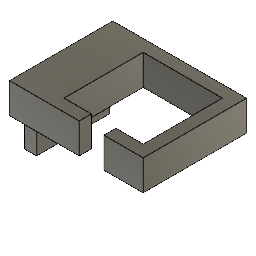
assembly v3 (Autodesk Fusion 360 archive; units mm, degrees)
design "holder_L"
Autodesk Fusion 360 part; units mm, degrees
sketch "Sketch1" plane through (0, 0, 0) normal (0, 0, 1) x (1, 0, 0)
  line L0 (0, 0) -> (13, 0)
  line L1 (13, 0) -> (13, 13)
  line L2 (13, 13) -> (0, 13)
  line L3 (0, 13) -> (0, 0)
  line L4 (-2, -2) -> (15, -2)
  line L5 (15, -2) -> (15, 15)
  line L6 (15, 15) -> (-2, 15)
  line L7 (-2, 15) -> (-2, -2)
  dimension "d1" = 13
  dimension "d2" = 13
  dimension "d3" = 2
  constraint horizontal L0
  constraint vertical L1
  constraint horizontal L2
  constraint vertical L3
  constraint coincident L0.start L3.end
  measures "d1" distance of L1.end L2.end
  measures "d2" distance of L0.end L1.end
extrude "Extrude1" add sketch "Sketch1" along normal blind 5
sketch "Sketch2" plane through (0, 0, 0) normal (0, 1, 0) x (-1, 0, 0)
  line L0 (-13, 0) -> (0, 0)
  line L1 (0, 0) -> (0, 5)
  line L2 (0, 5) -> (-13, 5)
  line L3 (-13, 5) -> (-13, 0)
  line L4 (-8.5, 5) -> (-4.5, 5)
  line L5 (-4.5, 5) -> (-4.5, 0)
  line L6 (-4.5, 0) -> (-8.5, 0)
  line L7 (-8.5, 0) -> (-8.5, 5)
  line L8 (-6.5, 0) -> (-6.5, 5)
  dimension "d6" = 4
  dimension "d7" = 90
  constraint horizontal L4
  constraint vertical L5
  constraint horizontal L6
  constraint vertical L7
  constraint coincident L0 L5.end
  constraint coincident L2 L4.start
  constraint midpoint L6 L8.start
  constraint midpoint L2 L8.end
  measures "d6" distance of L4.start L4.end
  measures "d7" angle of L4 L8
extrude "Extrude2" cut sketch "Sketch2" against normal blind 10 contours L0 L2 L4 L6 L7 L8 | L0 L2 L4 L5 L6 L8
extrude "Extrude3" add 1 faces at (-2, 9.3333, 1.6667) along direction (-1, 0, 0) blind 5
sketch "Sketch3" plane through (0, 0, 0) normal (0, 0, -1) x (1, 0, 0)
  line L0 (8.5, 2) -> (8.5, 0)
  line L1 (8.5, 0) -> (13, 0)
  line L2 (13, 0) -> (13, -13)
  line L3 (13, -13) -> (0, -13)
  line L4 (0, -13) -> (0, 0)
  line L5 (0, 0) -> (4.5, 0)
  line L6 (4.5, 0) -> (4.5, 2)
  line L7 (4.5, 2) -> (-7, 2)
  line L8 (-7, 2) -> (-7, -15)
  line L9 (-7, -15) -> (15, -15)
  line L10 (15, -15) -> (15, 2)
  line L11 (15, 2) -> (8.5, 2)
  line L12 (-7, 2) -> (-5, 2)
  line L13 (-5, 2) -> (-5, -15)
  line L14 (-5, -15) -> (-7, -15)
  line L15 (-7, -15) -> (-7, 2)
  dimension "d12" = 2
  constraint horizontal L12
  constraint vertical L13
  constraint horizontal L14
  constraint vertical L15
  constraint coincident L9 L13.end
  constraint coincident L7.end L8.start
  measures "d12" distance of L7.end L12.end
extrude "Extrude4" add sketch "Sketch3" along normal blind 6 contours L7 L8 L9 L12 L13 L14 L15
sketch "Sketch4" plane through (-5, 0, 0) normal (1, 0, 0) x (0, 1, 0)
  line L0 (15, 0) -> (-2, 0)
  line L1 (-2, 0) -> (-2, -6)
  line L2 (-2, -6) -> (15, -6)
  line L3 (15, -6) -> (15, 0)
  line L4 (-2, -2) -> (15, -2)
  circle A0 centre (3.5, -2) radius 1.5
  circle A1 centre (9.5, -2) radius 1.5
  line L5 (3.5, -2) -> (9.5, -2)
  line L6 (6.5, -2) -> (6.5, 0)
  dimension "d15" = 2
  dimension "d16" = 3
  dimension "d17" = 3
  dimension "d18" = 6
  dimension "d19" = 90
  constraint coincident L1 L4.start
  constraint coincident L3 L4.end
  constraint perpendicular L3 L4
  constraint coincident L4 A0.centre
  constraint coincident L4 A1.centre
  constraint coincident A0.centre L5.start
  constraint coincident A1.centre L5.end
  constraint midpoint L5 L6.start
  constraint midpoint L0 L6.end
  measures "d15" distance of L0 L4
  measures "d16" diameter of A0
  measures "d17" diameter of A1
  measures "d18" distance of A0.centre A1.centre
  measures "d19" angle of L0 L6
extrude "Extrude5" cut sketch "Sketch4" against normal blind 5 contours L4 A1 L5 | L4 A1 L5 | L4 A0 L5 | L4 A0 L5
sketch "Sketch5" plane through (-5, 0, 0) normal (1, 0, 0) x (0, 1, 0)
  circle A0 centre (3.5, -2) radius 1.5
  circle A1 centre (9.5, -2) radius 1.5
  line L0 (15, 0) -> (-2, 0)
  line L1 (-2, 0) -> (-2, -6)
  line L2 (-2, -6) -> (15, -6)
  line L3 (15, -6) -> (15, 0)
  line L4 (0.5, 0) -> (12.5, 0)
  line L5 (12.5, 0) -> (12.5, -6)
  line L6 (12.5, -6) -> (0.5, -6)
  line L7 (0.5, -6) -> (0.5, 0)
  line L8 (-2, -6) -> (15, -6)
  line L9 (15, -6) -> (15, 0)
  line L10 (15, 0) -> (-2, 0)
  line L11 (-2, 0) -> (-2, -6)
  dimension "d22" = 3
  dimension "d23" = 3
  constraint horizontal L4
  constraint vertical L5
  constraint horizontal L6
  constraint vertical L7
  constraint coincident L2 L5.end
  constraint coincident L0 L4.start
  constraint horizontal L8
  constraint vertical L9
  constraint horizontal L10
  constraint vertical L11
  constraint coincident L0.start L3.end
  constraint coincident L1.end L2.start
  measures "d22" distance of A0.centre L7
  measures "d23" distance of A1.centre L5
extrude "Extrude6" cut sketch "Sketch5" against normal blind 5 contours L0 L2 L3 L5 L8 L9 L10 | L0 L1 L2 L7 L8 L10 L11

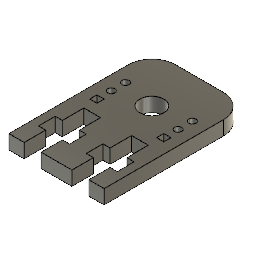
design "stand_L"
Autodesk Fusion 360 part; units mm, degrees
sketch "Sketch1" plane through (0, 0, 0) normal (0, 0, 1) x (1, 0, 0)
  line L0 (0, 0) -> (40, 0)
  line L1 (40, 0) -> (40, 60)
  line L2 (40, 60) -> (0, 60)
  line L3 (0, 60) -> (0, 0)
  line L4 (20, 60) -> (20, 27.089)
  circle A0 centre (20, 40) radius 5
  line L5 (6.5, 0) -> (13.5, 0)
  line L6 (13.5, 0) -> (13.5, 25)
  line L7 (13.5, 25) -> (6.5, 25)
  line L8 (6.5, 25) -> (6.5, 0)
  line L9 (26.5, 0) -> (33.5, 0)
  line L10 (33.5, 0) -> (33.5, 25)
  line L11 (33.5, 25) -> (26.5, 25)
  line L12 (26.5, 25) -> (26.5, 0)
  line L13 (10, 25) -> (30, 25)
  line L14 (20, 25) -> (20, 0)
  line L15 (0, 16) -> (40, 16)
  line L16 (3.5, 16) -> (16.5, 16)
  line L17 (16.5, 16) -> (16.5, 9)
  line L18 (16.5, 9) -> (3.5, 9)
  line L19 (3.5, 9) -> (3.5, 16)
  line L20 (3.5, 12.5) -> (6.5, 12.5)
  line L21 (10, 9) -> (10, 0)
  line L22 (23.5, 16) -> (23.5, 9)
  line L23 (23.5, 9) -> (36.5, 9)
  line L24 (36.5, 9) -> (36.5, 16)
  dimension "d1" = 40
  dimension "d2" = 60
  dimension "d3" = 10
  dimension "d4" = 40
  dimension "d5" = 7
  dimension "d6" = 7
  dimension "d7" = 25
  dimension "d8" = 25
  dimension "d9" = 20
  dimension "d10" = 90
  dimension "d11" = 90
  dimension "d12" = 13
  dimension "d13" = 90
  dimension "d14" = 7
  constraint horizontal L0
  constraint vertical L1
  constraint horizontal L2
  constraint vertical L3
  constraint coincident L0.start L3.end
  constraint midpoint L2 L4.start
  constraint perpendicular L2 L4
  constraint coincident L4 A0.centre
  constraint horizontal L5
  constraint vertical L6
  constraint horizontal L7
  constraint vertical L8
  constraint coincident L0 L5.start
  constraint horizontal L9
  constraint vertical L10
  constraint horizontal L11
  constraint vertical L12
  constraint coincident L0 L9.start
  constraint midpoint L7 L13.start
  constraint midpoint L11 L13.end
  constraint midpoint L13 L14.start
  constraint midpoint L0 L14.end
  constraint coincident L3 L15.start
  constraint coincident L1 L15.end
  constraint perpendicular L1 L15
  constraint horizontal L16
  constraint vertical L17
  constraint horizontal L18
  constraint vertical L19
  constraint coincident L15 L16.start
  constraint midpoint L19 L20.start
  constraint midpoint L8 L20.end
  constraint midpoint L18 L21.start
  constraint midpoint L5 L21.end
  constraint symmetric L14 L16.start L24.end
  constraint symmetric L14 L16.end L22.start
  constraint symmetric L14 L17.end L22.end
  constraint symmetric L14 L18.end L23.end
  measures "d1" distance of L0.start L0.end
  measures "d2" distance of L0.end L1.end
  measures "d3" diameter of A0
  measures "d4" distance of L0 A0.centre
  measures "d5" distance of L6.end L7.end
  measures "d6" distance of L10.end L11.end
  measures "d7" distance of L5.start L7.end
  measures "d8" distance of L9.end L10.end
  measures "d9" distance of L13.start L13.end
  measures "d10" angle of L0 L14
  measures "d11" angle of L8 L20
  measures "d12" distance of L17.end L18.end
  measures "d13" angle of L18 L21 L9.start
  measures "d14" distance of L16.end L17.end
extrude "Extrude1" add sketch "Sketch1" along normal blind 6 contours L0 L3 L8 L15 L18 L19 | L1 L2 L3 L7 L8 L10 L11 L13 L15 L16 | L0 L6 L14 L15 L17 L18 | L0 L12 L14 L15 L22 L23 | L6 L13 L14 L15 L16 | L12 L13 L14 L15 | L0 L1 L10 L15 L23 L24
sketch "Sketch2" plane through (0, 0, 6) normal (0, 0, 1) x (-1, 0, 0)
  circle A0 centre (-20, -40) radius 5
  line L0 (-33.5, 0) -> (-40, 0)
  line L1 (-40, 0) -> (-40, -60)
  line L2 (-40, -60) -> (0, -60)
  line L3 (0, -60) -> (0, 0)
  line L4 (0, 0) -> (-6.5, 0)
  line L5 (-6.5, 0) -> (-6.5, -9)
  line L6 (-6.5, -9) -> (-3.5, -9)
  line L7 (-3.5, -9) -> (-3.5, -16)
  line L8 (-3.5, -16) -> (-6.5, -16)
  line L9 (-6.5, -16) -> (-6.5, -25)
  line L10 (-6.5, -25) -> (-13.5, -25)
  line L11 (-13.5, -25) -> (-13.5, -16)
  line L12 (-13.5, -16) -> (-16.5, -16)
  line L13 (-16.5, -16) -> (-16.5, -9)
  line L14 (-16.5, -9) -> (-13.5, -9)
  line L15 (-13.5, -9) -> (-13.5, 0)
  line L16 (-13.5, 0) -> (-26.5, 0)
  line L17 (-26.5, 0) -> (-26.5, -9)
  line L18 (-26.5, -9) -> (-23.5, -9)
  line L19 (-23.5, -9) -> (-23.5, -16)
  line L20 (-23.5, -16) -> (-26.5, -16)
  line L21 (-26.5, -16) -> (-26.5, -25)
  line L22 (-26.5, -25) -> (-33.5, -25)
  line L23 (-33.5, -25) -> (-33.5, -16)
  line L24 (-33.5, -16) -> (-36.5, -16)
  line L25 (-36.5, -16) -> (-36.5, -9)
  line L26 (-36.5, -9) -> (-33.5, -9)
  line L27 (-33.5, -9) -> (-33.5, 0)
  line L28 (0, -40) -> (-40, -40)
  line L29 (-6, -45) -> (-6, -35)
  circle A1 centre (-6, -43) radius 1.5
  circle A2 centre (-6, -37) radius 1.5
  line L30 (-6, -43) -> (-6, -37)
  line L31 (-6, -40) -> (0, -40)
  line L32 (-20, -40) -> (-20, -45)
  circle A3 centre (-34, -43) radius 1.5
  circle A4 centre (-34, -37) radius 1.5
  dimension "d17" = 6
  dimension "d18" = 3
  dimension "d19" = 3
  dimension "d20" = 6
  dimension "d21" = 90
  constraint coincident L3 L28.start
  constraint coincident L1 L28.end
  constraint perpendicular L1 L28
  constraint perpendicular L28 L29
  constraint coincident L29 A1.centre
  constraint coincident L29 A2.centre
  constraint coincident A1.centre L30.start
  constraint coincident A2.centre L30.end
  constraint midpoint L30 L31.start
  constraint coincident A0.centre L32.start
  constraint coincident A0 L32.end
  constraint vertical L32
  constraint coincident L28 A0.centre
  constraint symmetric A1 L32 A3
  constraint symmetric A2 L32 A4
  measures "d17" distance of L3 L29
  measures "d18" diameter of A1
  measures "d19" diameter of A2
  measures "d20" distance of A1.centre A2.centre
  measures "d21" angle of L3 L31
extrude "Extrude2" cut sketch "Sketch2" against normal blind 5 contours L29 A1 L30 | L29 A1 L30 | L29 A2 L30 | L29 A2 L30 | A3 | A4
sketch "Sketch3" plane through (0, 0, 6) normal (0, 0, 1) x (-1, 0, 0)
  circle A0 centre (-6, -37) radius 1.5
  circle A1 centre (-34, -43) radius 1.5
  circle A2 centre (-6, -43) radius 1.5
  circle A3 centre (-34, -37) radius 1.5
  circle A4 centre (-20, -40) radius 5
  line L0 (-33.5, 0) -> (-40, 0)
  line L1 (-40, 0) -> (-40, -60)
  line L2 (-40, -60) -> (0, -60)
  line L3 (0, -60) -> (0, 0)
  line L4 (0, 0) -> (-6.5, 0)
  line L5 (-6.5, 0) -> (-6.5, -9)
  line L6 (-6.5, -9) -> (-3.5, -9)
  line L7 (-3.5, -9) -> (-3.5, -16)
  line L8 (-3.5, -16) -> (-6.5, -16)
  line L9 (-6.5, -16) -> (-6.5, -25)
  line L10 (-6.5, -25) -> (-13.5, -25)
  line L11 (-13.5, -25) -> (-13.5, -16)
  line L12 (-13.5, -16) -> (-16.5, -16)
  line L13 (-16.5, -16) -> (-16.5, -9)
  line L14 (-16.5, -9) -> (-13.5, -9)
  line L15 (-13.5, -9) -> (-13.5, 0)
  line L16 (-13.5, 0) -> (-26.5, 0)
  line L17 (-26.5, 0) -> (-26.5, -9)
  line L18 (-26.5, -9) -> (-23.5, -9)
  line L19 (-23.5, -9) -> (-23.5, -16)
  line L20 (-23.5, -16) -> (-26.5, -16)
  line L21 (-26.5, -16) -> (-26.5, -25)
  line L22 (-26.5, -25) -> (-33.5, -25)
  line L23 (-33.5, -25) -> (-33.5, -16)
  line L24 (-33.5, -16) -> (-36.5, -16)
  line L25 (-36.5, -16) -> (-36.5, -9)
  line L26 (-36.5, -9) -> (-33.5, -9)
  line L27 (-33.5, -9) -> (-33.5, 0)
  line L28 (0, -31) -> (-40, -31)
  line L29 (-4.5, -32.5) -> (-7.5, -32.5)
  line L30 (-7.5, -32.5) -> (-7.5, -29.5)
  line L31 (-7.5, -29.5) -> (-4.5, -29.5)
  line L32 (-4.5, -29.5) -> (-4.5, -32.5)
  line L33 (-6, -37) -> (0, -37)
  line L34 (-6, -37) -> (-6, -32.5)
  line L35 (-4.5, -31) -> (0, -31)
  line L36 (-20, -40) -> (-20, -43)
  line L37 (-35.5, -32.5) -> (-32.5, -32.5)
  line L38 (-32.5, -32.5) -> (-32.5, -29.5)
  line L39 (-35.5, -29.5) -> (-35.5, -32.5)
  line L40 (-32.5, -29.5) -> (-35.5, -29.5)
  dimension "d24" = 3
  dimension "d25" = 3
  dimension "d26" = 90
  dimension "d27" = 6
  dimension "d28" = 90
  constraint coincident L3 L28.start
  constraint coincident L1 L28.end
  constraint perpendicular L1 L28
  constraint horizontal L29
  constraint vertical L30
  constraint horizontal L31
  constraint vertical L32
  constraint coincident A0.centre L33.start
  constraint coincident L3 L33.end
  constraint perpendicular L3 L33
  constraint midpoint L29 L34.end
  constraint midpoint L32 L35.start
  constraint coincident A4.centre L36.start
  constraint vertical L36
  constraint symmetric L29.start L36 L37.start
  constraint symmetric L29.end L36 L37.end
  constraint symmetric L30.end L36 L38.end
  constraint symmetric L31.end L36 L39.start
  measures "d24" distance of L29.end L30.end
  measures "d25" distance of L30.end L31.end
  measures "d26" angle of L29 L34
  measures "d27" distance of L28 L33
  measures "d28" angle of L32 L35
extrude "Extrude3" cut sketch "Sketch3" against normal blind 5 contours L28 L29 L30 L32 | L28 L30 L31 L32 | L28 L37 L38 L39 | L28 L38 L39 L40
fillet "Fillet1" radius 10 1 edges at (0, 60, 3)
fillet "Fillet2" radius 10 1 edges at (40, 60, 3)
extrude "Extrude4" cut 6 faces at (6.8158, 43.2169, 1) (6.1827, 37.4654, 1) (5.5, 31.5, 1) (33.5, 30.5, 1) (33.9601, 37.4654, 1) (33.2997, 43.1474, 1) along direction (0, 0, -1) blind 5

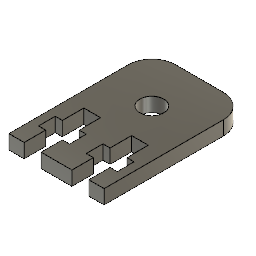
design "stand_R"
Autodesk Fusion 360 part; units mm, degrees
sketch "Sketch1" plane through (0, 0, 0) normal (0, 0, 1) x (1, 0, 0)
  line L0 (0, 0) -> (40, 0)
  line L1 (40, 0) -> (40, 60)
  line L2 (40, 60) -> (0, 60)
  line L3 (0, 60) -> (0, 0)
  line L4 (20, 60) -> (20, 27.089)
  circle A0 centre (20, 40) radius 5
  line L5 (6.5, 0) -> (13.5, 0)
  line L6 (13.5, 0) -> (13.5, 25)
  line L7 (13.5, 25) -> (6.5, 25)
  line L8 (6.5, 25) -> (6.5, 0)
  line L9 (26.5, 0) -> (33.5, 0)
  line L10 (33.5, 0) -> (33.5, 25)
  line L11 (33.5, 25) -> (26.5, 25)
  line L12 (26.5, 25) -> (26.5, 0)
  line L13 (10, 25) -> (30, 25)
  line L14 (20, 25) -> (20, 0)
  line L15 (0, 16) -> (40, 16)
  line L16 (3.5, 16) -> (16.5, 16)
  line L17 (16.5, 16) -> (16.5, 9)
  line L18 (16.5, 9) -> (3.5, 9)
  line L19 (3.5, 9) -> (3.5, 16)
  line L20 (3.5, 12.5) -> (6.5, 12.5)
  line L21 (10, 9) -> (10, 0)
  line L22 (23.5, 16) -> (23.5, 9)
  line L23 (23.5, 9) -> (36.5, 9)
  line L24 (36.5, 9) -> (36.5, 16)
  dimension "d1" = 40
  dimension "d2" = 60
  dimension "d3" = 10
  dimension "d4" = 40
  dimension "d5" = 7
  dimension "d6" = 7
  dimension "d7" = 25
  dimension "d8" = 25
  dimension "d9" = 20
  dimension "d10" = 90
  dimension "d11" = 90
  dimension "d12" = 13
  dimension "d13" = 90
  dimension "d14" = 7
  constraint horizontal L0
  constraint vertical L1
  constraint horizontal L2
  constraint vertical L3
  constraint coincident L0.start L3.end
  constraint midpoint L2 L4.start
  constraint perpendicular L2 L4
  constraint coincident L4 A0.centre
  constraint horizontal L5
  constraint vertical L6
  constraint horizontal L7
  constraint vertical L8
  constraint coincident L0 L5.start
  constraint horizontal L9
  constraint vertical L10
  constraint horizontal L11
  constraint vertical L12
  constraint coincident L0 L9.start
  constraint midpoint L7 L13.start
  constraint midpoint L11 L13.end
  constraint midpoint L13 L14.start
  constraint midpoint L0 L14.end
  constraint coincident L3 L15.start
  constraint coincident L1 L15.end
  constraint perpendicular L1 L15
  constraint horizontal L16
  constraint vertical L17
  constraint horizontal L18
  constraint vertical L19
  constraint coincident L15 L16.start
  constraint midpoint L19 L20.start
  constraint midpoint L8 L20.end
  constraint midpoint L18 L21.start
  constraint midpoint L5 L21.end
  constraint symmetric L14 L16.start L24.end
  constraint symmetric L14 L16.end L22.start
  constraint symmetric L14 L17.end L22.end
  constraint symmetric L14 L18.end L23.end
  measures "d1" distance of L0.start L0.end
  measures "d2" distance of L0.end L1.end
  measures "d3" diameter of A0
  measures "d4" distance of L0 A0.centre
  measures "d5" distance of L6.end L7.end
  measures "d6" distance of L10.end L11.end
  measures "d7" distance of L5.start L7.end
  measures "d8" distance of L9.end L10.end
  measures "d9" distance of L13.start L13.end
  measures "d10" angle of L0 L14
  measures "d11" angle of L8 L20
  measures "d12" distance of L17.end L18.end
  measures "d13" angle of L18 L21 L9.start
  measures "d14" distance of L16.end L17.end
extrude "Extrude1" add sketch "Sketch1" along normal blind 6 contours L0 L3 L8 L15 L18 L19 | L1 L2 L3 L7 L8 L10 L11 L13 L15 L16 | L0 L6 L14 L15 L17 L18 | L0 L12 L14 L15 L22 L23 | L6 L13 L14 L15 L16 | L12 L13 L14 L15 | L0 L1 L10 L15 L23 L24
fillet "Fillet1" radius 10 1 edges at (0, 60, 3)
fillet "Fillet2" radius 10 1 edges at (40, 60, 3)

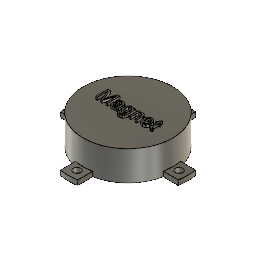
design "cap"
Autodesk Fusion 360 part; units mm, degrees
sketch "Sketch1" plane through (0, 0, 0) normal (0, 0, 1) x (1, 0, 0)
  circle A0 centre (0, 0) radius 16
  circle A1 centre (0, 0) radius 18
  dimension "d1" = 32
  dimension "d2" = 2
  constraint coincident A0.centre A1.centre
  constraint concentric A0 A1
  measures "d1" diameter of A0
  measures "d2" distance of A0 A1
extrude "Extrude1" add sketch "Sketch1" along normal blind 10
sketch "Sketch2" plane through (0, 0, 10) normal (0, 0, 1) x (-1, 0, 0)
  circle A0 centre (0, 0) radius 16
  circle A1 centre (0, 0) radius 18
  circle A2 centre (0, 0) radius 18
  constraint coincident A0.centre A1.centre
  constraint tangent A1 A2
extrude "Extrude2" add sketch "Sketch2" along normal blind 2 contours A0 | A1 A2
sketch "Sketch3" plane through (0, 0, 0) normal (0, 0, -1) x (1, 0, 0)
  circle A0 centre (0, 0) radius 16
  circle A1 centre (0, 0) radius 18
  line L0 (-3.5, 24) -> (3.5, 24)
  line L1 (3.5, 24) -> (3.5, -27)
  line L2 (3.5, -27) -> (-3.5, -27)
  line L3 (-3.5, -27) -> (-3.5, 24)
  line L4 (0, 0) -> (0, 18)
  line L5 (0, 18) -> (0, 24)
  circle A2 centre (0, 20.5) radius 1.5
  line L6 (0, 19) -> (0.9, 19)
  circle A3 centre (0, 0) radius 24
  line L7 (27, -3.5) -> (-24, -3.5)
  line L8 (-24, 3.5) -> (27, 3.5)
  circle A4 centre (-20.5, 0) radius 1.5
  line L9 (3.5, 27) -> (3.5, -24)
  line L10 (-3.5, -24) -> (-3.5, 27)
  circle A5 centre (0, -20.5) radius 1.5
  line L11 (-27, 3.5) -> (24, 3.5)
  line L12 (24, -3.5) -> (-27, -3.5)
  circle A6 centre (20.5, 0) radius 1.5
  dimension "d7" = 7
  dimension "d8" = 90
  dimension "d9" = 3
  dimension "d10" = 1
  dimension "d11" = 3.5
  dimension "d13" = 360
  constraint horizontal L0
  constraint vertical L1
  constraint horizontal L2
  constraint vertical L3
  constraint coincident A0.centre A1.centre
  constraint coincident A1 L4.end
  constraint parallel L1 L4
  constraint midpoint L0 L5.end
  constraint coincident L5 A2.centre
  constraint coincident A2 L6.start
  constraint coincident L5 L6.start
  constraint tangent A2 L6
  constraint coincident L5.end A3
  measures "d7" distance of L0.start L0.end
  measures "d8" angle of L0 L5
  measures "d9" diameter of A2
  measures "d10" distance of L4.end L6.start
  measures "d11" distance of L0 A2.centre
extrude "Extrude3" add sketch "Sketch3" against normal blind 3 contours A1 A3 L7 L8 L11 L12 | A1 L1 L5 A2 A3 L9 | A1 L1 L3 A3 L9 L10 | A1 L3 L5 A2 A3 L10 | A1 A3 L7 L8 L11 L12
extrude "Extrude4" cut 4 faces at (2.8333, -20.6333, 3) (-20.6707, 2.8319, 3) (20.6707, -2.8319, 3) (-2.8333, 20.6333, 3) along direction (0, 0, -1) blind 1
sketch "Sketch4" plane through (0, 0, 12) normal (0, 0, 1) x (-1, 0, 0)
  circle A0 centre (0, 0) radius 18
  line L0 (11, 2) -> (-11, 2) construction
  line L1 (-11, 2) -> (-11, -3) construction
  line L2 (-11, -3) -> (11, -3) construction
  line L3 (11, -3) -> (11, 2) construction
  dimension "d18" = 5
  text T0 "Magnet" font "Arial" height 5 align left top in box 22 x 5 at (11, 2) x (-1, 0) y (0, -1) spacing 1 kerned
extrude "Extrude5" add sketch "Sketch4" along normal blind 1 text T0

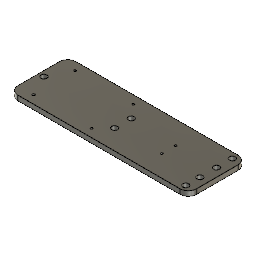
design "base"
Autodesk Fusion 360 part; units mm, degrees
sketch "Sketch1" plane through (0, 0, 0) normal (0, 0, 1) x (1, 0, 0)
  line L0 (10, 0) -> (205, 0)
  line L1 (215, 10) -> (215, 60)
  line L2 (205, 70) -> (10, 70)
  line L3 (0, 60) -> (0, 10)
  arc A0 (10, 70) -> (0, 60) centre (10, 60) ccw
  arc A1 (0, 10) -> (10, 0) centre (10, 10) ccw
  arc A2 (215, 60) -> (205, 70) centre (205, 60) ccw
  arc A3 (205, 0) -> (215, 10) centre (205, 10) ccw
  line L4 (205, 70) -> (205, 0)
  circle A4 centre (205, 43.9323) radius 3.5
  circle A5 centre (205, 23.9323) radius 3.5
  line L5 (102.5, 70) -> (102.5, 0)
  line L6 (205, 43.9323) -> (102.5, 43.9323)
  line L7 (205, 23.9323) -> (102.5, 23.9323)
  circle A6 centre (102.5, 43.9323) radius 3.5
  circle A7 centre (102.5, 23.9323) radius 3.5
  line L8 (89, 60) -> (49, 60)
  line L9 (49, 60) -> (49, 10)
  line L10 (49, 10) -> (89, 10)
  line L11 (89, 10) -> (89, 60)
  line L12 (102.5, 35) -> (89, 35)
  line L13 (49, 52.5466) -> (19, 52.5466)
  line L14 (19, 52.5466) -> (19, 17.4534)
  line L15 (19, 17.4534) -> (49, 17.4534)
  line L16 (49, 17.4534) -> (49, 52.5466)
  line L17 (19, 35) -> (49, 35)
  line L18 (0, 0) -> (0, 24.1752)
  line L19 (0, 0) -> (-15.0158, 0)
  line L20 (89, 60) -> (19, 60)
  line L21 (19, 60) -> (19, 10)
  line L22 (19, 10) -> (89, 10)
  line L23 (89, 10) -> (89, 60)
  circle A8 centre (89, 60) radius 1.25
  circle A9 centre (89, 10) radius 1.25
  circle A10 centre (19, 10) radius 1.5
  circle A11 centre (19, 60) radius 1.25
  point P0 (215, 0)
  point P1 (215, 70)
  point P2 (0, 70)
  dimension "d1" = 215
  dimension "d2" = 70
  dimension "d3" = 10
  dimension "d4" = 10
  dimension "d5" = 10
  dimension "d6" = 10
  dimension "d7" = 10
  dimension "d8" = 7
  dimension "d9" = 7
  dimension "d10" = 20
  dimension "d11" = 102.5
  dimension "d12" = 7
  dimension "d13" = 7
  dimension "d14" = 40
  dimension "d15" = 50
  dimension "d16" = 90
  dimension "d17" = 13.5
  dimension "d18" = 30
  dimension "d19" = 90
  dimension "d20" = 2.5
  dimension "d21" = 2.5
  dimension "d22" = 3
  dimension "d23" = 2.5
  constraint horizontal L0
  constraint vertical L1
  constraint horizontal L2
  constraint vertical L3
  constraint coincident P2 L2
  constraint coincident P2 L3
  constraint tangent L2 A0
  constraint tangent L3 A0
  constraint tangent L0 A1
  constraint tangent L3 A1
  constraint coincident P1 L1
  constraint coincident P1 L2
  constraint tangent L1 A2
  constraint tangent L2 A2
  constraint coincident P0 L0
  constraint coincident P0 L1
  constraint tangent L0 A3
  constraint tangent L1 A3
  constraint coincident L2 A2.end
  constraint coincident L0 A3.start
  constraint perpendicular L0 L4
  constraint coincident L4 A4.centre
  constraint coincident L4 A5.centre
  constraint coincident L2 L5.start
  constraint coincident L0 L5.end
  constraint perpendicular L0 L5
  constraint coincident A4.centre L6.start
  constraint coincident L5 L6.end
  constraint perpendicular L5 L6
  constraint coincident A5.centre L7.start
  constraint coincident L5 L7.end
  constraint perpendicular L5 L7
  constraint coincident L6.end A6.centre
  constraint coincident L7.end A7.centre
  constraint horizontal L8
  constraint vertical L9
  constraint horizontal L10
  constraint vertical L11
  constraint midpoint L5 L12.start
  constraint midpoint L11 L12.end
  constraint horizontal L13
  constraint vertical L14
  constraint horizontal L15
  constraint vertical L16
  constraint coincident L9 L13.start
  constraint midpoint L14 L17.start
  constraint midpoint L9 L17.end
  constraint coincident L18.start L19.start
  constraint vertical L18
  constraint perpendicular L18 L19
  constraint coincident L3 L18.end
  constraint horizontal L20
  constraint vertical L21
  constraint horizontal L22
  constraint vertical L23
  constraint collinear L14 L21
  constraint coincident L8.start L11.end
  constraint coincident L10.end L11.start
  constraint coincident L21.end L22.start
  constraint coincident L20.end L21.start
  measures "d1" distance of P1 P2
  measures "d2" distance of P0 P1
  measures "d3" radius of A0
  measures "d4" radius of A1
  measures "d5" radius of A2
  measures "d6" radius of A3
  measures "d7" distance of L1 L4
  measures "d8" diameter of A5
  measures "d9" diameter of A4
  measures "d10" distance of A4.centre A5.centre
  measures "d11" distance of L4 L5
  measures "d12" diameter of A6
  measures "d13" diameter of A7
  measures "d14" distance of L8.start L8.end
  measures "d15" distance of L8.start L10.end
  measures "d16" angle of L5 L12
  measures "d17" distance of L7.end L11
  measures "d18" distance of L13.start L13.end
  measures "d19" angle of L16 L17
  measures "d20" diameter of A8
  measures "d21" diameter of A9
  measures "d22" diameter of A10
  measures "d23" diameter of A11
extrude "Extrude1" add sketch "Sketch1" along normal blind 6 contours L0 L2 L3 A0 A1 L5 A6 A7 L18 | L0 L4 A5 L5 L7 A7 | L1 A2 A3 L4 A4 A5 | L4 A4 A5 L5 L6 L7 A6 A7 | L2 L4 A4 L5 L6 A6 | L8 L9 L10 L11 L16 L20 L22 L23 A8 A9 | L9 L13 L20 L21 A11 | L9 L13 L14 L16 L17 L21 | L9 L14 L15 L16 L17 L21 | L9 L15 L21 L22 A10
sketch "Sketch2" plane through (0, 0, 6) normal (0, 0, 1) x (-1, 0, 0)
  circle A0 centre (-19, -60) radius 1.25
  circle A1 centre (-102.5, -43.9323) radius 3.5
  circle A2 centre (-89, -60) radius 1.25
  circle A3 centre (-89, -10) radius 1.25
  circle A4 centre (-102.5, -23.9323) radius 3.5
  circle A5 centre (-19, -10) radius 1.5
  circle A6 centre (-205, -23.9323) radius 3.5
  circle A7 centre (-205, -43.9323) radius 3.5
  arc A8 (0, -10) -> (-10, 0) centre (-10, -10) ccw
  line L0 (-10, 0) -> (-205, 0)
  arc A9 (-205, 0) -> (-215, -10) centre (-205, -10) ccw
  line L1 (-215, -10) -> (-215, -60)
  arc A10 (-215, -60) -> (-205, -70) centre (-205, -60) ccw
  line L2 (-205, -70) -> (-10, -70)
  arc A11 (-10, -70) -> (0, -60) centre (-10, -60) ccw
  line L3 (0, -60) -> (0, -10)
  line L4 (-157.5, -70) -> (-157.5, 0)
  line L5 (-102.5, -43.9323) -> (-102.5, -23.9323)
  circle A12 centre (-157.5, -42.1823) radius 1.25
  circle A13 centre (-157.5, -25.6823) radius 1.25
  line L6 (-151.1278, -40.9323) -> (-166.7652, -40.9323)
  line L7 (-166.7652, -40.9323) -> (-166.7652, -26.9323)
  line L8 (-166.7652, -26.9323) -> (-151.1278, -26.9323)
  line L9 (-151.1278, -26.9323) -> (-151.1278, -40.9323)
  line L10 (-151.1278, -33.9323) -> (-102.5, -33.9323)
  dimension "d26" = 55
  dimension "d27" = 14
  dimension "d28" = 90
  dimension "d29" = 2.5
  dimension "d30" = 2.5
  constraint coincident L2 L4.start
  constraint coincident L0 L4.end
  constraint perpendicular L0 L4
  constraint coincident A1.centre L5.start
  constraint coincident A4.centre L5.end
  constraint coincident L4 A12.centre
  constraint coincident L4 A13.centre
  constraint horizontal L6
  constraint vertical L7
  constraint horizontal L8
  constraint vertical L9
  constraint tangent A12 L6
  constraint tangent A13 L8
  constraint midpoint L9 L10.start
  constraint midpoint L5 L10.end
  measures "d26" distance of L4 L5
  measures "d27" distance of L6.end L7.end
  measures "d28" angle of L5 L10
  measures "d29" diameter of A12
  measures "d30" diameter of A13
extrude "Extrude2" cut sketch "Sketch2" against normal blind 5 contours L4 A13 | L4 A13 | L4 A12 | L4 A12
sketch "Sketch3" plane through (0, 0, 6) normal (0, 0, 1) x (-1, 0, 0)
  circle A0 centre (-157.5, -42.1823) radius 1.25
  circle A1 centre (-157.5, -25.6823) radius 1.25
  circle A2 centre (-205, -43.9323) radius 3.5
  circle A3 centre (-19, -10) radius 1.5
  circle A4 centre (-89, -60) radius 1.25
  circle A5 centre (-89, -10) radius 1.25
  circle A6 centre (-102.5, -43.9323) radius 3.5
  circle A7 centre (-19, -60) radius 1.25
  circle A8 centre (-205, -23.9323) radius 3.5
  circle A9 centre (-102.5, -23.9323) radius 3.5
  arc A10 (0, -10) -> (-10, 0) centre (-10, -10) ccw
  line L0 (-10, 0) -> (-205, 0)
  arc A11 (-205, 0) -> (-215, -10) centre (-205, -10) ccw
  line L1 (-215, -10) -> (-215, -60)
  arc A12 (-215, -60) -> (-205, -70) centre (-205, -60) ccw
  line L2 (-205, -70) -> (-10, -70)
  arc A13 (-10, -70) -> (0, -60) centre (-10, -60) ccw
  line L3 (0, -60) -> (0, -10)
  line L4 (-6.5, -60) -> (-6.5, -10)
  circle A14 centre (-6.5, -35) radius 3.5
  line L5 (-10, -60) -> (-10, -10)
  line L6 (-6.5, -35) -> (0, -35)
  line L7 (-205, -70) -> (-205, 0)
  circle A15 centre (-205, -63) radius 3.5
  circle A16 centre (-205, -7) radius 3.5
  dimension "d33" = 7
  dimension "d36" = 7
  dimension "d37" = 7
  dimension "d38" = 7
  dimension "d39" = 7
  constraint perpendicular L0 L4
  constraint midpoint L4 A14.centre
  constraint coincident A13.centre L5.start
  constraint coincident A10.centre L5.end
  constraint tangent A14 L5
  constraint coincident A14.centre L6.start
  constraint midpoint L3 L6.end
  constraint perpendicular L3 L6
  constraint coincident L2 A12.end
  constraint coincident L0 A11.start
  constraint perpendicular L0 L7
  constraint coincident L7 A15.centre
  constraint coincident L7 A16.centre
  constraint coincident A2.centre L7
  measures "d33" diameter of A14
  measures "d36" diameter of A15
  measures "d37" diameter of A16
  measures "d38" distance of L2 A15.centre
  measures "d39" distance of L0 A16.centre
extrude "Extrude3" cut sketch "Sketch3" against normal blind 7 contours L7 A15 | L7 A15 | L7 A16 | L7 A16 | L4 A14 | L4 A14 L6 | L4 A14 L6
extrude "Extrude4" cut 1 faces at (157.8221, 41.8565, 1) along direction (0, 0, -1) blind 5
extrude "Extrude5" cut 1 faces at (157.1946, 25.2747, 1) along direction (0, 0, -1) blind 5

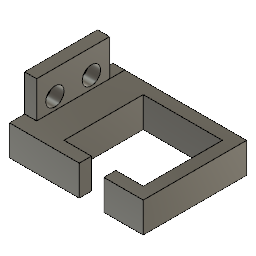
design "holder_R"
Autodesk Fusion 360 part; units mm, degrees
sketch "Sketch1" plane through (0, 0, 0) normal (0, 0, 1) x (1, 0, 0)
  line L0 (0, 0) -> (13, 0)
  line L1 (13, 0) -> (13, 13)
  line L2 (13, 13) -> (0, 13)
  line L3 (0, 13) -> (0, 0)
  line L4 (-2, -2) -> (15, -2)
  line L5 (15, -2) -> (15, 15)
  line L6 (15, 15) -> (-2, 15)
  line L7 (-2, 15) -> (-2, -2)
  dimension "d1" = 13
  dimension "d2" = 13
  dimension "d3" = 2
  constraint horizontal L0
  constraint vertical L1
  constraint horizontal L2
  constraint vertical L3
  constraint coincident L0.start L3.end
  measures "d1" distance of L1.end L2.end
  measures "d2" distance of L0.end L1.end
extrude "Extrude1" add sketch "Sketch1" along normal blind 5
sketch "Sketch2" plane through (0, 0, 0) normal (0, 1, 0) x (-1, 0, 0)
  line L0 (-13, 0) -> (0, 0)
  line L1 (0, 0) -> (0, 5)
  line L2 (0, 5) -> (-13, 5)
  line L3 (-13, 5) -> (-13, 0)
  line L4 (-8.5, 5) -> (-4.5, 5)
  line L5 (-4.5, 5) -> (-4.5, 0)
  line L6 (-4.5, 0) -> (-8.5, 0)
  line L7 (-8.5, 0) -> (-8.5, 5)
  line L8 (-6.5, 0) -> (-6.5, 5)
  dimension "d6" = 4
  dimension "d7" = 90
  constraint horizontal L4
  constraint vertical L5
  constraint horizontal L6
  constraint vertical L7
  constraint coincident L0 L5.end
  constraint coincident L2 L4.start
  constraint midpoint L6 L8.start
  constraint midpoint L2 L8.end
  measures "d6" distance of L4.start L4.end
  measures "d7" angle of L4 L8
extrude "Extrude2" cut sketch "Sketch2" against normal blind 10 contours L0 L2 L4 L6 L7 L8 | L0 L2 L4 L5 L6 L8
extrude "Extrude3" add 1 faces at (-2, 9.3333, 1.6667) along direction (-1, 0, 0) blind 5
sketch "Sketch3" plane through (0, 0, 0) normal (0, 0, -1) x (1, 0, 0)
  line L0 (8.5, 2) -> (8.5, 0)
  line L1 (8.5, 0) -> (13, 0)
  line L2 (13, 0) -> (13, -13)
  line L3 (13, -13) -> (0, -13)
  line L4 (0, -13) -> (0, 0)
  line L5 (0, 0) -> (4.5, 0)
  line L6 (4.5, 0) -> (4.5, 2)
  line L7 (4.5, 2) -> (-7, 2)
  line L8 (-7, 2) -> (-7, -15)
  line L9 (-7, -15) -> (15, -15)
  line L10 (15, -15) -> (15, 2)
  line L11 (15, 2) -> (8.5, 2)
  line L12 (-7, 2) -> (-5, 2)
  line L13 (-5, 2) -> (-5, -15)
  line L14 (-5, -15) -> (-7, -15)
  line L15 (-7, -15) -> (-7, 2)
  dimension "d12" = 2
  constraint horizontal L12
  constraint vertical L13
  constraint horizontal L14
  constraint vertical L15
  constraint coincident L9 L13.end
  constraint coincident L7.end L8.start
  measures "d12" distance of L7.end L12.end
extrude "Extrude4" add sketch "Sketch3" along normal blind 6 contours L7 L8 L9 L12 L13 L14 L15
sketch "Sketch4" plane through (-5, 0, 0) normal (1, 0, 0) x (0, 1, 0)
  line L0 (15, 0) -> (-2, 0)
  line L1 (-2, 0) -> (-2, -6)
  line L2 (-2, -6) -> (15, -6)
  line L3 (15, -6) -> (15, 0)
  line L4 (-2, -2) -> (15, -2)
  circle A0 centre (3.5, -2) radius 1.5
  circle A1 centre (9.5, -2) radius 1.5
  line L5 (3.5, -2) -> (9.5, -2)
  line L6 (6.5, -2) -> (6.5, 0)
  dimension "d15" = 2
  dimension "d16" = 3
  dimension "d17" = 3
  dimension "d18" = 6
  dimension "d19" = 90
  constraint coincident L1 L4.start
  constraint coincident L3 L4.end
  constraint perpendicular L3 L4
  constraint coincident L4 A0.centre
  constraint coincident L4 A1.centre
  constraint coincident A0.centre L5.start
  constraint coincident A1.centre L5.end
  constraint midpoint L5 L6.start
  constraint midpoint L0 L6.end
  measures "d15" distance of L0 L4
  measures "d16" diameter of A0
  measures "d17" diameter of A1
  measures "d18" distance of A0.centre A1.centre
  measures "d19" angle of L0 L6
extrude "Extrude5" cut sketch "Sketch4" against normal blind 5 contours L4 A1 L5 | L4 A1 L5 | L4 A0 L5 | L4 A0 L5
mirror "Mirror1" about plane through (-2, 15, 5) normal (0, 0, 1) of bodies 1 merged
sketch "Sketch5" plane through (15, 0, 0) normal (1, 0, 0) x (0, 1, 0)
  line L0 (-2, 0) -> (15, 0)
  line L1 (15, 0) -> (15, 10)
  line L2 (15, 10) -> (-2, 10)
  line L3 (-2, 10) -> (-2, 0)
  line L4 (-15, 5) -> (21, 5)
  line L5 (21, 5) -> (21, -10.6123)
  line L6 (21, -10.6123) -> (-15, -10.6123)
  line L7 (-15, -10.6123) -> (-15, 5)
  constraint horizontal L4
  constraint vertical L5
  constraint horizontal L6
  constraint vertical L7
extrude "Extrude6" cut sketch "Sketch5" against normal blind 100 contours L0 L1 L3 L4 | L0 L1 L3 L4 L5 L6 L7
sketch "Sketch6" plane through (-5, 0, 0) normal (1, 0, 0) x (0, 1, 0)
  circle A0 centre (3.5, 12) radius 1.5
  circle A1 centre (9.5, 12) radius 1.5
  line L0 (-2, 10) -> (15, 10)
  line L1 (15, 10) -> (15, 16)
  line L2 (15, 16) -> (-2, 16)
  line L3 (-2, 16) -> (-2, 10)
  line L4 (-2, 16) -> (0.5, 16)
  line L5 (0.5, 16) -> (0.5, 10)
  line L6 (0.5, 10) -> (-2, 10)
  line L7 (-2, 10) -> (-2, 16)
  line L8 (15, 16) -> (12.5, 16)
  line L9 (12.5, 16) -> (12.5, 10)
  line L10 (12.5, 10) -> (15, 10)
  line L11 (15, 10) -> (15, 16)
  dimension "d26" = 3
  dimension "d27" = 3
  constraint horizontal L4
  constraint vertical L5
  constraint horizontal L6
  constraint vertical L7
  constraint coincident L0 L5.end
  constraint coincident L2.end L3.start
  constraint horizontal L8
  constraint vertical L9
  constraint horizontal L10
  constraint vertical L11
  constraint coincident L0 L9.end
  constraint coincident L1.end L2.start
  measures "d26" distance of A0.centre L5
  measures "d27" distance of A1.centre L9
extrude "Extrude7" cut sketch "Sketch6" against normal blind 6 contours L0 L2 L3 L4 L5 L6 L7 | L0 L1 L2 L8 L9 L10 L11
